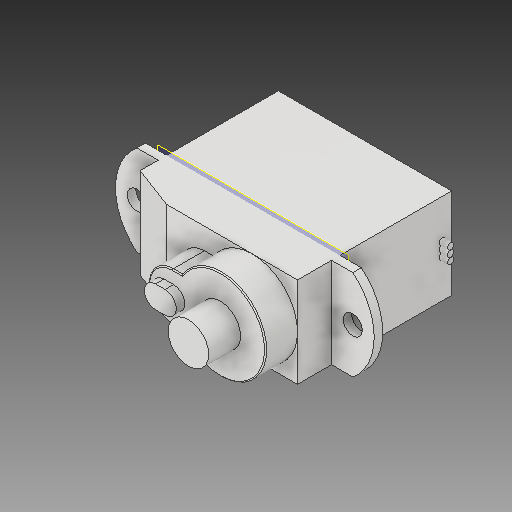
# Autodesk Inventor part: Servo
Saved by Autodesk Inventor 2018.1 (Build 221171000, 171)
## iProperties
Part Number: Servo
Material: 一般
Document SubType Name: Modeling
Designer: sktom
Density: 1 g/cm^3
Appearance: 滑らか - 白
Author: sktom
Autodesk Inventor part; units mm, degrees
ref_plane "YZ Plane" through (0, 0, 0) normal (1, 0, 0) x (0, 1, 0)
ref_plane "XZ Plane" through (0, 0, 0) normal (0, 1, 0) x (-1, 0, 0)
ref_plane "XY Plane" through (0, 0, 0) normal (0, 0, 1) x (1, 0, 0)
sketch "スケッチ1" plane through (0, 0, 0) normal (0, 0, 1) x (1, 0, 0)
  line L0 (-8.15, -4.25) -> (8.15, -4.25)
  line L1 (8.15, -4.25) -> (8.15, 4.25)
  line L2 (8.15, 4.25) -> (-8.15, 4.25)
  line L3 (-8.15, 4.25) -> (-8.15, -4.25)
  line L4 (-8.15, -4.25) -> (8.15, 4.25) construction
  line L5 (8.15, -4.25) -> (-8.15, 4.25) construction
  point P0 (0, 0)
  dimension "d0" = 16.3
  dimension "d1" = 8.5
  constraints: 12 end point, 2 midpoint, 2 parallel, 1 horizontal, 1 perpendicular
  measures "d0" distance of L1.end L2.end
  measures "d1" distance of L0.end L1.end
extrude "押し出し1" add sketch "スケッチ1" along normal blind 14.5
ref_plane "作業平面2" through (0, 0, 10.5) normal (0, 0, -1) x (-1, 0, 0)
sketch "スケッチ3" plane through (0, 0, 10.5) normal (0, 0, -1) x (-1, 0, 0)
  circle A0 centre (10.15, 0) radius 0.9
  line L0 (8.15, 4.25) -> (8.15, -4.25) projected
  line L1 (8.15, -4.25) -> (8.15, 4.25)
  line L2 (8.15, 4.25) -> (10.15, 4.25)
  line L3 (8.15, -4.25) -> (10.15, -4.25)
  line L4 (8.15, 4.25) -> (8.15, -4.25) projected
  arc A1 (10.15, -4.25) -> (10.15, 4.25) centre (6.6589, 0) ccw
  point P0 (0, 0)
  point P1 (8.15, 0)
  dimension "d11" = 1.8
  dimension "d12" = 2
  dimension "d13" = 5.5
  constraints: 6 end point, 2 centre point, 2 point on circle, 2 vertical alignment, 1 collinear, 1 horizontal, 1 horizontal alignment, 1 midpoint, 1 perpendicular
  measures "d11" diameter of A0
  measures "d12" distance from line of L0 A0.centre
  measures "d13" radius of A1
extrude "押し出し3" add sketch "スケッチ3" against normal blind 0.8
mirror "ミラー1" about plane through (0, 0, 0) normal (1, 0, 0) of "押し出し3"
sketch "スケッチ4" plane through (8.15, -4.25, 0) normal (1, 0, 0) x (0, 0, -1)
  circle A0 centre (-0.9, 4.25) radius 0.3
  circle A1 centre (-0.9, 4.85) radius 0.3
  circle A2 centre (-0.9, 3.65) radius 0.3
  line L0 (0, 0) -> (0, 8.5) projected
  point P0 (0, 4.25)
  point P1 (0, 4.25)
  dimension "d16" = 0.6
  dimension "d18" = 0.9
  constraints: 4 equal radius, 3 centre point, 2 vertical alignment, 1 horizontal alignment, 1 midpoint
  measures "d16" diameter of A1
  measures "d18" distance of point (0, 4.25) A0.centre
extrude "押し出し4" add sketch "スケッチ4" along normal blind 0.8
chamfer "面取り1" distance 4 distance2 1.5 1 edges at (-8.15, 0, 14.5) measured on face at (-7.65, 0, 14.5)
sketch "スケッチ5" plane through (0, 0, 10.5) normal (0, 0, -1) x (-1, 0, 0)
  point P0 (0, 0)
sketch "スケッチ6" plane through (0, 0, 14.5) normal (0, 0, 1) x (1, 0, 0)
  arc A0 (0.2944, -2.25) -> (0.2944, 2.25) centre (3.9, 0) ccw
  line L0 (8.15, 4.25) -> (-4.15, 4.25) projected
  line L1 (8.15, -4.25) -> (8.15, 4.25) projected
  line L2 (-4.15, -4.25) -> (8.15, -4.25) projected
  arc A1 (-0.6, 2.25) -> (-0.6, -2.25) centre (-0.6, 0) ccw
  line L3 (-0.6, 2.25) -> (0.2944, 2.25)
  line L4 (-0.6, -2.25) -> (0.2944, -2.25)
  point P0 (0, 0)
  dimension "d24" = 4.5
  dimension "d25" = 4.5
  constraints: 5 tangent, 4 end point, 4 point on circle, 2 centre point, 1 horizontal, 1 horizontal alignment, 1 parallel
  measures "d24" distance of A0.centre A1.centre
  measures "d25" diameter of A1
extrude "押し出し5" add sketch "スケッチ6" along normal blind 3 contours L4 A1 L3 A0
sketch "スケッチ7" plane through (0, 0, 17.5) normal (0, 0, 1) x (1, 0, 0)
  arc A0 (8.15, 0) -> (3.9, 4.25) centre (3.9, 0) ccw projected
  circle A1 centre (3.9, 0) radius 1.9
  point P0 (0, 0)
  dimension "d28" = 3.8
  constraints: 1 centre point, 1 coincident
  measures "d28" diameter of A1
extrude "押し出し6" add sketch "スケッチ7" along normal blind 3
sketch "スケッチ8" plane through (0, 0, 17.5) normal (0, 0, 1) x (1, 0, 0)
  line L0 (-1.4, 0) -> (-0.5, 0) construction
  line L1 (-1.4, -1.05) -> (-0.5, -1.05)
  line L2 (-0.5, 1.05) -> (-1.4, 1.05)
  arc A0 (-1.4, 1.05) -> (-1.4, -1.05) centre (-1.4, 0) ccw
  arc A1 (-0.5, -1.05) -> (-0.5, 1.05) centre (-0.5, 0) ccw
  arc A2 (-0.6, 2.25) -> (-0.6, -2.25) centre (-0.6, 0) ccw projected
  point P0 (0, 0)
  point P1 (-0.95, 0)
  dimension "d31" = 2.1
  dimension "d32" = 3
  dimension "d33" = 0.8
  constraints: 8 end point, 4 point on circle, 4 tangent, 2 centre point, 1 horizontal, 1 horizontal alignment, 1 midpoint, 1 parallel
  measures "d31" distance between parallel lines of L1 L2
  measures "d33" distance of A2.centre L0.start
extrude "押し出し7" add sketch "スケッチ8" along normal blind 0.8
fillet "フィレット1" radius 0.1 4 edges at (8.15, 0, 17.5) (-2.85, 0, 17.5) (-0.1528, 2.25, 17.5) (-0.1528, -2.25, 17.5)
